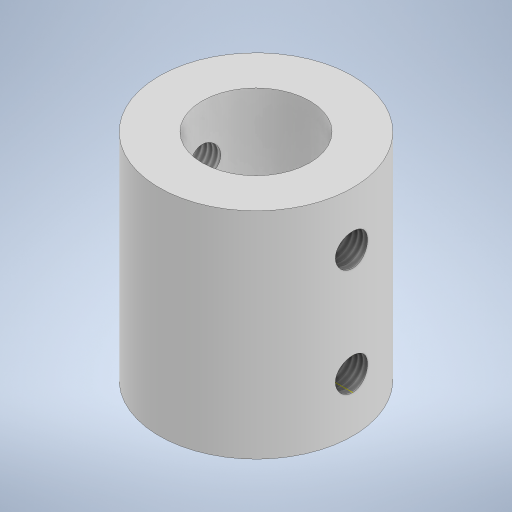
# Autodesk Inventor part: Втулка энкодер
Saved by Autodesk Inventor 2023 (Build 270158000, 158)
## iProperties
Created: 2022-04-28
Part Number: Втулка энкодер
Material: Типовые
Document SubType Name: Modeling
Designer: User
Density: 1 g/cm^3
Appearance: По умолчанию
Author: User
Autodesk Inventor part; units mm, degrees
ref_plane "YZ Plane" through (0, 0, 0) normal (1, 0, 0) x (0, 1, 0)
ref_plane "XZ Plane" through (0, 0, 0) normal (0, 1, 0) x (-1, 0, 0)
ref_plane "XY Plane" through (0, 0, 0) normal (0, 0, 1) x (1, 0, 0)
sketch "Эскиз1" plane through (0, 0, 0) normal (0, 1, 0) x (-1, 0, 0)
  circle A0 centre (0, 0) radius 3.5
  circle A1 centre (0, 0) radius 9
  dimension "d0" = 7
  dimension "d1" = 18
  constraints: 2 centre point, 2 coincident
  measures "d0" diameter of A0
  measures "d1" diameter of A1
extrude "Выдавливание1" add sketch "Эскиз1" along normal blind 20
sketch "Эскиз2" plane through (0, 20, 0) normal (0, 1, 0) x (1, 0, 0)
  circle A0 centre (0, 0) radius 5
  dimension "d4" = 10
  constraints: 1 centre point, 1 coincident
  measures "d4" diameter of A0
extrude "Выдавливание2" cut sketch "Эскиз2" against normal blind 10
sketch "Эскиз3" plane through (0, 0, 0) normal (1, 0, 0) x (0, 1, 0)
  line L0 (20, -9) -> (20, 9) projected
  line L1 (20, 0) -> (15, 0)
  line L2 (0, 0) -> (5, 0)
  circle A0 centre (15, 0) radius 1.5
  circle A1 centre (5, 0) radius 1.5
  dimension "d7" = 5
  dimension "d8" = 5
  dimension "d9" = 3
  dimension "d10" = 3
  constraints: 4 end point, 2 centre point, 2 coincident, 1 horizontal, 1 midpoint, 1 point on line
  measures "d7" distance of L1.start L1.end
  measures "d8" distance of L2.start L2.end
  measures "d9" diameter of A0
  measures "d10" diameter of A1
extrude "Выдавливание3" cut sketch "Эскиз3" along normal mid plane 27.5
thread "Резьба1" size "M3x0.5" class "6H" standard "ISO Metric profile" full length
thread "Резьба2" size "M3x0.5" class "6H" standard "ISO Metric profile" full length
sketch "Эскиз4" plane through (0, 0, 0) normal (0, 0, 1) x (1, 0, 0)
  line L0 (3.5, 10) -> (3.5, 0) projected
  line L1 (-5, 10) -> (5, 10) projected
  line L2 (-3.5, 10) -> (-3.5, 0) projected
  line L3 (-9, 6.5) -> (-3.5, 6.5) projected
  line L4 (-9, 3.5) -> (-3.5, 3.5) projected
  line L5 (3.5, 3.5) -> (9, 3.5) projected
  line L6 (3.5, 6.5) -> (9, 6.5) projected
  line L7 (-3.5, 5) -> (3.5, 5)
  line L8 (0, 5) -> (0, 0)
  constraints: 4 end point, 3 midpoint, 1 vertical
